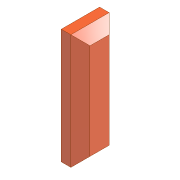
# Autodesk Inventor part: Print_Parts_U
Saved by Autodesk Inventor 2020.1 (Build 241239000, 239)
## iProperties
Created: 2020-10-06
Part Number: Print_Parts_U
Material: PC/ABS プラスチック
Document SubType Name: Modeling
Designer: kenta iguchi
Density: 0.357273 g/cm^3
Appearance: 滑らか - 淡いオレンジ
Author: kenta iguchi
Autodesk Inventor part; units mm, degrees
ref_plane "YZ Plane" through (0, 0, 0) normal (1, 0, 0) x (0, 1, 0)
ref_plane "XZ Plane" through (0, 0, 0) normal (0, 1, 0) x (-1, 0, 0)
ref_plane "XY Plane" through (0, 0, 0) normal (0, 0, 1) x (1, 0, 0)
sketch "スケッチ2" plane through (0, 0, 0) normal (1, 0, 0) x (0, 1, 0)
  line L0 (-30, 10) -> (30, 10)
  line L1 (30, 10) -> (30, -10)
  line L2 (30, -10) -> (-30, -10)
  line L3 (-30, -10) -> (-30, 10)
  line L4 (-30, 10) -> (30, -10) construction
  line L5 (30, 10) -> (-30, -10) construction
  point P0 (0, 0)
  dimension "d4" = 60
  dimension "d5" = 20
  constraints: 12 end point, 2 midpoint, 2 parallel, 1 horizontal, 1 perpendicular
  measures "d4" distance of L1.end L2.end
  measures "d5" distance of L0.end L1.end
extrude "押し出し2" add sketch "スケッチ2" along normal blind 10
chamfer "面取り1" distance 5 angle 45 4 edges at (10, 0, -10) (10, 30, 0) (10, 0, 10) (10, -30, 0)
